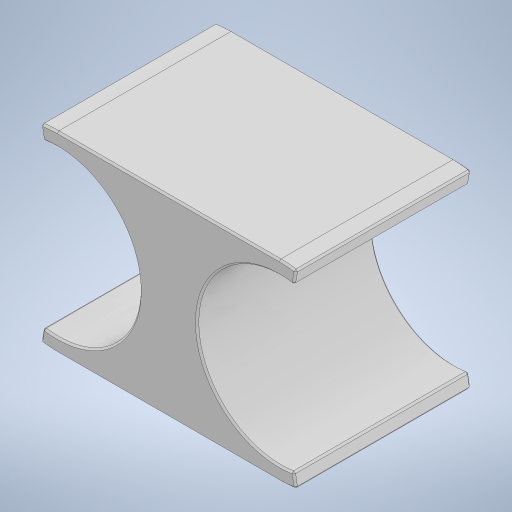
# Autodesk Inventor part: two-sided-01
Saved by Autodesk Inventor 2023.1 (Build 271208000, 208)
## iProperties
Created: 2023-04-07
Part Number: two-sided-01
Material: Generic
Document SubType Name: Modeling
Designer: caleb
Density: 1 g/cm^3
Appearance: Default
Author: caleb
Autodesk Inventor part; units mm, degrees
ref_plane "YZ Plane" through (0, 0, 0) normal (1, 0, 0) x (0, 1, 0)
ref_plane "XZ Plane" through (0, 0, 0) normal (0, 1, 0) x (-1, 0, 0)
ref_plane "XY Plane" through (0, 0, 0) normal (0, 0, 1) x (1, 0, 0)
sketch "Sketch2" plane through (0, 0, 0) normal (0, 0, 1) x (1, 0, 0)
  arc A0 (-18.496, -13.695) -> (-18.496, 13.695) centre (-16.0813, 0) ccw
  arc A1 (-18.1487, -11.7254) -> (-18.1487, 11.7254) centre (-16.0813, 0) ccw
  line L0 (-16.0813, 0) -> (-18.496, 13.695) construction
  line L1 (-16.0813, 0) -> (-18.496, -13.695) construction
  line L2 (-18.496, 13.695) -> (-18.1487, 11.7254)
  line L3 (-18.496, -13.695) -> (-18.1487, -11.7254)
  line L4 (4.175, 13.9062) -> (4.175, -13.9062)
  line L5 (4.175, 13.9062) -> (-16.0813, 13.9062)
  line L6 (4.175, -13.9062) -> (-16.0812, -13.9063)
  line L7 (-2.175, 13.9062) -> (-2.175, -13.9062) construction
  line L8 (-4.175, 0) -> (4.175, 0) construction
  point P0 (0, 0)
  point P1 (0, 0)
  point P2 (0, 0)
  dimension "d3" = 160
  dimension "d4" = 11.9062
  dimension "d5" = 2
  dimension "d8" = 6.35
  constraints: 18 end point, 7 point on circle, 3 collinear, 3 tangent, 2 centre point, 2 coincident, 2 midpoint, 2 point on line, 2 vertical, 1 horizontal, 1 horizontal alignment, 1 parallel, 1 vertical alignment
  measures "d3" angle of L1 L0
  measures "d4" radius of A1
  measures "d5" radial gap between concentric circles of A0 A1
  measures "d8" distance between parallel lines of L4 L7
extrude "Extrusion1" add sketch "Sketch2" against normal blind 25.4
mirror "Mirror2" about plane through (0, 0, 0) normal (1, 0, 0) of "Extrusion1"
chamfer "Chamfer1" distance 0.25 angle 45 32 edges at (-4.175, 0, 0) (-18.496, -13.695, -12.7) (-18.1487, -11.7254, -12.7) (18.496, -13.695, -12.7) (18.1487, -11.7254, -12.7) (4.175, 0, 0) (18.1487, 11.7254, -12.7) (4.175, 0, -25.4) (-4.175, 0, -25.4) (-18.496, 13.695, -12.7) (-18.1487, 11.7254, -12.7) (0, 13.9062, 0) (-17.2933, 13.8533, 0) (17.2933, 13.8533, 0) (-18.3224, 12.7102, 0) (18.3224, 12.7102, 0) (18.3224, -12.7102, 0) (-17.2933, -13.8533, 0) (0, -13.9063, 0) (17.2933, -13.8533, 0) (-18.3224, -12.7102, 0) (-18.3224, -12.7102, -25.4) (-17.2933, -13.8533, -25.4) (0, -13.9063, -25.4) (17.2933, -13.8533, -25.4) (18.3224, -12.7102, -25.4) (18.3224, 12.7102, -25.4) (18.496, 13.695, -12.7) (0, 13.9062, -25.4) (17.2933, 13.8533, -25.4) (-17.2933, 13.8533, -25.4) (-18.3224, 12.7102, -25.4)
ref_plane "Work Plane3" through (0, 0, 0) normal (1, 0, 0) x (0, 1, 0)
equation "\"d3\" = angle"
equation "\"d5\" = thickness"
equation "\"angle\" = 160deg"
equation "\"thickness\" = 2"
body "Solid2"
